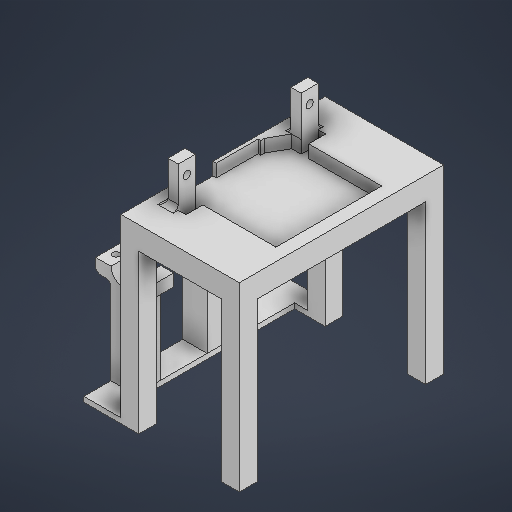
# Autodesk Inventor part: OMG_20kg_servo_side_profile(0.4mm)
Saved by Autodesk Inventor 2026.1 (Build 301233020, 233B)
## iProperties
Created: 2026-02-21
Part Number: OMG_20kg_servo_side_profile(0.4mm)
Material: Generic
Document SubType Name: Modeling
Designer: Lars
Density: 1 g/cm^3
Appearance: Default
Author: Lars
Autodesk Inventor part; units mm, degrees
ref_plane "YZ Plane" through (0, 0, 0) normal (1, 0, 0) x (0, 1, 0)
ref_plane "XZ Plane" through (0, 0, 0) normal (0, 1, 0) x (-1, 0, 0)
ref_plane "XY Plane" through (0, 0, 0) normal (0, 0, 1) x (1, 0, 0)
sketch "Sketch1" plane through (0, 0, 0) normal (0, 1, 0) x (-1, 0, 0)
  line L0 (0, 0) -> (28.63, 0)
  line L1 (28.63, 0) -> (28.63, -41.25) construction
  line L2 (28.63, -41.25) -> (0, -41.25)
  line L3 (0, -41.25) -> (0, 0)
  line L4 (28.63, 6.675) -> (31.43, 6.675)
  line L5 (31.43, 6.675) -> (31.43, 0)
  line L6 (31.43, -47.925) -> (28.63, -47.925)
  line L7 (28.63, -47.925) -> (28.63, -41.25)
  line L8 (31.43, -20.625) -> (28.63, -20.625) construction
  line L9 (38.98, 0) -> (31.43, 0)
  line L10 (31.43, 0) -> (31.43, -41.25) construction
  line L11 (31.43, -41.25) -> (35.18, -41.25)
  line L12 (38.98, -41.25) -> (38.98, -34.5) construction
  line L13 (31.43, -41.25) -> (35.18, -41.25) construction
  line L14 (38.98, 0) -> (38.98, -1) construction
  line L15 (38.98, -34.5) -> (35.18, -41.25)
  line L16 (38.98, -34.5) -> (38.98, -33)
  line L17 (35.18, -41.25) -> (38.98, -41.25) construction
  line L18 (38.98, 0) -> (38.98, -1) construction
  line L19 (38.98, -1) -> (39.98, -1)
  line L20 (39.98, -1) -> (39.98, -4)
  line L21 (39.98, -33) -> (38.98, -33)
  line L22 (38.98, -33) -> (38.98, -1) construction
  line L23 (38.98, -1) -> (38.98, -33) construction
  line L24 (38.98, -33) -> (38.98, -34.5) construction
  line L25 (38.98, -1) -> (38.98, 0)
  line L26 (38.98, -33) -> (38.98, -1) construction
  line L27 (31.43, 0) -> (31.43, -41.25) construction
  line L28 (31.43, -41.25) -> (31.43, -47.925)
  line L29 (28.63, -41.25) -> (28.63, 0) construction
  line L30 (28.63, 0) -> (28.63, 6.675)
  line L31 (28.63, 0) -> (31.43, 0) construction
  line L32 (31.43, -41.25) -> (28.63, -41.25) construction
  line L33 (39.98, -1) -> (39.98, -4) construction
  line L34 (39.98, -4) -> (41.28, -4)
  line L35 (41.28, -4) -> (41.28, -16.6)
  line L36 (41.28, -16.6) -> (39.98, -16.6)
  line L37 (39.98, -16.6) -> (39.98, -4) construction
  line L38 (39.98, -4) -> (39.98, -16.6) construction
  line L39 (39.98, -16.6) -> (39.98, -33)
  line L40 (41.38, -16.7) -> (41.38, -3.9)
  line L41 (41.38, -3.9) -> (40.08, -3.9)
  line L42 (40.08, -3.9) -> (40.08, -0.9)
  line L43 (40.08, -0.9) -> (39.08, -0.9)
  line L44 (39.08, -0.9) -> (39.08, 0.1)
  line L45 (39.08, 0.1) -> (31.53, 0.1)
  line L46 (31.53, 0.1) -> (31.53, 6.775)
  line L47 (31.53, 6.775) -> (28.53, 6.775)
  line L48 (28.53, 6.775) -> (28.53, 0.1)
  line L49 (28.53, 0.1) -> (-0.1, 0.1)
  line L50 (-0.1, 0.1) -> (-0.1, -41.35)
  line L51 (-0.1, -41.35) -> (28.53, -41.35)
  line L52 (28.53, -41.35) -> (28.53, -48.025)
  line L53 (28.53, -48.025) -> (31.53, -48.025)
  line L54 (31.53, -48.025) -> (31.53, -41.35)
  line L55 (31.53, -41.35) -> (35.2385, -41.35)
  line L56 (35.2385, -41.35) -> (39.08, -34.5262)
  line L57 (39.08, -34.5262) -> (39.08, -33.1)
  line L58 (39.08, -33.1) -> (40.08, -33.1)
  line L59 (40.08, -33.1) -> (40.08, -16.7)
  line L60 (40.08, -16.7) -> (41.38, -16.7)
  line L61 (0, -20.625) -> (39.98, -20.625) construction
  line L62 (44.99, 9.375) -> (-5.01, 9.375)
  line L63 (-5.01, 9.375) -> (-5.01, -50.625)
  line L64 (-5.01, -50.625) -> (44.99, -50.625)
  line L65 (44.99, -50.625) -> (44.99, 9.375)
  line L66 (19.99, 9.375) -> (19.99, -50.625) construction
  point P0 (30.03, 6.675)
  point P1 (19.99, -20.625)
  dimension "d0" = 28.63
  dimension "d1" = 41.25
  dimension "d2" = 2.8
  dimension "d3" = 54.6
  dimension "d4" = 7.55
  dimension "d5" = 41.25
  dimension "d6" = 3.75
  dimension "d7" = 34.5
  dimension "d8" = 1
  dimension "d9" = 32
  dimension "d10" = 1
  dimension "d11" = 6.675
  dimension "d12" = 3
  dimension "d13" = 1.3
  dimension "d14" = 12.6
  dimension "d15" = 0.1
  dimension "d16" = 50
  dimension "d17" = 60
  constraints: 134 end point, 35 parallel, 17 perpendicular, 8 midpoint, 7 horizontal, 5 vertical, 1 point on line, 20 other
  measures "d0" distance of L1.end L2.end
  measures "d1" distance of L0.end L1.end
  measures "d2" distance of L6.start L6.end
  measures "d3" distance of L4.end L6.start
  measures "d4" distance of L12.start L10.end
  measures "d5" distance of L12.start L9.start
  measures "d6" distance of L10.end L11.end
  measures "d7" distance of L9.start L12.end
  measures "d8" distance of L9.start L14.end
  measures "d9" distance of L19.end L21.start
  measures "d10" distance of L21.start L16.end
  measures "d11" distance from line of point (30.03, 6.675) L31
  measures "d12" distance of L19.end L20.end
  measures "d13" distance of L35.end L36.end
  measures "d14" distance of L34.end L35.end
  measures "d15" distance between parallel lines of L35 L40
  measures "d16" distance of L64.end L63.end
  measures "d17" distance of L63.end L62.end
extrude "Extrusion1" add sketch "Sketch1" along normal blind 5 contours L65 L64 L63 L62
sketch "Sketch3" plane through (5.01, 0, -50.625) normal (0, 0, -1) x (-1, 0, 0)
  line L0 (0, 5) -> (50, 5) projected
  line L1 (0, 0) -> (50, 0) projected
  line L2 (0, 5) -> (50, 5)
  line L3 (50, 5) -> (50, 0)
  line L4 (50, 0) -> (0, 0)
  line L5 (0, 0) -> (0, 5)
  point P0 (5.01, 0)
  constraints: 8 end point, 2 parallel, 1 horizontal, 1 perpendicular
sketch "Sketch4" plane through (-44.99, 0, 9.375) normal (0, 0, 1) x (1, 0, 0)
  line L0 (0, 0) -> (0, 5) projected
  line L1 (50, 0) -> (0, 0) projected
  line L2 (0, 5) -> (50, 5)
  line L3 (50, 5) -> (50, 0)
  line L4 (50, 0) -> (0, 0)
  line L5 (0, 0) -> (0, 5)
  point P0 (44.99, 0)
  constraints: 8 end point, 2 parallel, 1 horizontal, 1 perpendicular
extrude "Extrusion2" add sketch "Sketch4" along normal blind 10
extrude "Extrusion3" add sketch "Sketch3" along normal blind 10
sketch "Sketch5" plane through (0, 5, 0) normal (0, 1, 0) x (1, 0, 0)
  line L0 (-41.38, 3.9) -> (-41.38, 16.7) projected
  line L1 (-44.99, -19.375) -> (-44.99, 60.625) projected
  line L2 (-44.99, 16.7) -> (-44.99, -19.375)
  line L3 (-44.99, -19.375) -> (-41.38, -19.375)
  line L4 (-41.38, -19.375) -> (-41.38, 16.7)
  line L5 (-44.99, 60.625) -> (-41.38, 60.625)
  line L6 (-41.38, 60.625) -> (-41.38, 16.7)
  line L7 (-44.99, 16.7) -> (-44.99, 60.625)
  point P0 (0, 0)
  constraints: 12 end point, 2 parallel, 1 horizontal, 1 perpendicular
extrude "Extrusion4" cut sketch "Sketch5" against normal blind 10
sketch "Sketch6" plane through (0, 0, 0) normal (0, -1, 0) x (1, 0, 0)
  line L0 (5.01, -60.625) -> (5.01, 19.375) projected
  line L1 (5.01, 19.375) -> (-41.3631, 19.375)
  line L2 (-41.3631, 19.375) -> (-41.3631, -60.625)
  line L3 (-41.3631, -60.625) -> (5.01, -60.625)
  line L4 (5.01, -60.625) -> (5.01, 19.375)
  point P0 (0, 0)
  constraints: 8 end point, 2 parallel, 1 horizontal, 1 perpendicular
extrude "Extrusion5" add sketch "Sketch6" along normal blind 4
sketch "Sketch7" plane through (0, 5, 0) normal (0, 1, 0) x (1, 0, 0)
  line L0 (-31.53, -0.1) -> (-39.08, -0.1) projected
  line L1 (-31.53, -0.1) -> (-35.53, -0.1)
  line L2 (-35.53, -0.1) -> (-35.53, -6.775)
  line L3 (-35.53, -6.775) -> (-31.53, -6.775)
  line L4 (-31.53, -6.775) -> (-31.53, -0.1)
  line L5 (-31.53, 41.3538) -> (-35.53, 41.3538)
  line L6 (-35.53, 41.3538) -> (-35.53, 48.025)
  line L7 (-35.53, 48.025) -> (-31.53, 48.025)
  line L8 (-31.53, 48.025) -> (-31.53, 41.3538)
  point P0 (0, 0)
  dimension "d28" = 4
  dimension "d29" = 4
  constraints: 16 end point, 4 parallel, 2 horizontal, 2 perpendicular, 1 point on line
  measures "d28" distance of L3.end L2.end
  measures "d29" distance of L6.end L7.end
extrude "Extrusion6" add sketch "Sketch7" along normal blind 15.7
sketch "Sketch8" plane through (-35.53, 5, 0.1) normal (-1, 0, 0) x (0, 0, 1)
  line L0 (6.675, 15.7) -> (0, 15.7) projected
  line L1 (3.3375, 15.7) -> (3.3375, 10.325) construction
  line L2 (-41.4538, 15.7) -> (-48.125, 15.7) projected
  line L3 (-44.7894, 15.7) -> (-44.7894, 10.325) construction
  circle A0 centre (-44.7894, 10.325) radius 1.45
  circle A1 centre (3.3375, 10.325) radius 1.45
  point P0 (-0.1, -5)
  dimension "d32" = 5.375
  dimension "d33" = 5.375
  dimension "d34" = 2.9
  dimension "d35" = 2.9
  constraints: 4 end point, 2 centre point, 2 coincident, 2 midpoint, 2 vertical
  measures "d32" distance of L1.start L1.end
  measures "d33" distance of L3.start L3.end
  measures "d34" diameter of A0
  measures "d35" diameter of A1
extrude "Extrusion7" cut sketch "Sketch8" against normal through all
fillet "Fillet1" radius 2 4 edges at (-35.53, 5, -44.6894) (-35.53, 5, 3.4375) (-33.53, 5, 6.775) (-33.53, 5, -48.025)
sketch "Sketch9" plane through (0, -4, 0) normal (0, -1, 0) x (1, 0, 0)
  line L0 (-41.38, -60.625) -> (5.01, -60.625) projected
  line L1 (-41.38, -60.625) -> (-34.38, -60.625)
  line L2 (-34.38, -60.625) -> (-34.38, -53.625)
  line L3 (-34.38, -53.625) -> (-41.38, -53.625)
  line L4 (-41.38, -53.625) -> (-41.38, -60.625)
  line L5 (5.01, -60.625) -> (-1.99, -60.625)
  line L6 (-1.99, -60.625) -> (-1.99, -53.625)
  line L7 (-1.99, -53.625) -> (5.01, -53.625)
  line L8 (5.01, -53.625) -> (5.01, -60.625)
  line L9 (5.01, 19.375) -> (-41.38, 19.375) projected
  line L10 (5.01, 19.375) -> (-1.99, 19.375)
  line L11 (-1.99, 19.375) -> (-1.99, 12.375)
  line L12 (-1.99, 12.375) -> (5.01, 12.375)
  line L13 (5.01, 12.375) -> (5.01, 19.375)
  line L14 (-41.38, 19.375) -> (-34.38, 19.375)
  line L15 (-34.38, 19.375) -> (-34.38, 12.375)
  line L16 (-34.38, 12.375) -> (-41.38, 12.375)
  line L17 (-41.38, 12.375) -> (-41.38, 19.375)
  point P0 (0, 0)
  dimension "d39" = 7
  dimension "d40" = 7
  dimension "d41" = 7
  dimension "d42" = 7
  dimension "d43" = 7
  dimension "d44" = 7
  dimension "d45" = 7
  dimension "d46" = 7
  constraints: 32 end point, 8 parallel, 4 horizontal, 4 perpendicular
  measures "d39" distance of L3.end L2.end
  measures "d40" distance of L2.end L1.end
  measures "d41" distance of L6.end L7.end
  measures "d42" distance of L5.end L6.end
  measures "d43" distance of L12.end L11.end
  measures "d44" distance of L11.end L10.end
  measures "d45" distance of L15.end L16.end
  measures "d46" distance of L14.end L15.end
extrude "Extrusion8" add sketch "Sketch9" along normal blind 60
sketch "Sketch10" plane through (0, -64, 0) normal (0, -1, 0) x (1, 0, 0)
  line L0 (5.01, -60.625) -> (5.01, 19.375) projected
  line L1 (5.01, 19.375) -> (-54.99, 19.375)
  line L2 (-54.99, 19.375) -> (-54.99, -60.625)
  line L3 (-54.99, -60.625) -> (5.01, -60.625)
  line L4 (5.01, -60.625) -> (5.01, 19.375)
  point P0 (0, 0)
  dimension "d49" = 60
  constraints: 8 end point, 2 parallel, 1 horizontal, 1 perpendicular
  measures "d49" distance of L3.end L2.end
extrude "Extrusion9" add sketch "Sketch10" along normal blind 2
sketch "Sketch12" plane through (0, -64, 0) normal (0, 1, 0) x (1, 0, 0)
  line L0 (-41.3631, 3.9) -> (-41.3631, 16.7) projected
  line L1 (-41.3631, 10.3) -> (-46.3231, 10.3) construction
  line L2 (-46.3231, 10.3) -> (-46.3231, 1.25) construction
  line L3 (-46.3231, 10.3) -> (-46.3231, 19.35) construction
  line L4 (-46.3231, 1.25) -> (-55.9231, 1.25)
  line L5 (-55.9231, 1.25) -> (-55.9231, -8.75)
  line L6 (-55.9231, -8.75) -> (-46.3231, -8.75)
  line L7 (-46.3231, -8.75) -> (-46.3231, 1.25)
  line L8 (-46.3231, 19.35) -> (-55.9231, 19.35)
  line L9 (-55.9231, 19.35) -> (-55.9231, 29.35)
  line L10 (-55.9231, 29.35) -> (-46.3231, 29.35)
  line L11 (-46.3231, 29.35) -> (-46.3231, 19.35)
  point P0 (0, 0)
  dimension "d52" = 4.96
  dimension "d53" = 9.05
  dimension "d54" = 9.05
  dimension "d55" = 9.6
  dimension "d56" = 10
  dimension "d57" = 9.6
  dimension "d58" = 10
  constraints: 22 end point, 4 parallel, 3 horizontal, 2 perpendicular, 2 vertical, 1 midpoint
  measures "d52" distance of L1.start L1.end
  measures "d53" distance of L1.end L2.end
  measures "d54" distance of L1.end L3.end
  measures "d55" distance of L6.end L5.end
  measures "d56" distance of L5.end L4.end
  measures "d57" distance of L9.end L10.end
  measures "d58" distance of L8.end L9.end
extrude "Extrusion10" add sketch "Sketch12" along normal blind 38.85
sketch "Sketch14" plane through (-55.9231, -64, -29.35) normal (-1, 0, 0) x (0, 0, 1)
  line L0 (0, 0) -> (0, 38.85) projected
  line L1 (10, 0) -> (10, 38.85) projected
  line L2 (0, 38.85) -> (10, 38.85)
  line L3 (10, 38.85) -> (10, 33.85)
  line L4 (10, 33.85) -> (0, 33.85)
  line L5 (0, 33.85) -> (0, 38.85)
  line L6 (28.1, 0) -> (28.1, 38.85) projected
  line L7 (38.1, 0) -> (38.1, 38.85) projected
  line L8 (28.1, 38.85) -> (38.1, 38.85)
  line L9 (38.1, 38.85) -> (38.1, 33.85)
  line L10 (38.1, 33.85) -> (28.1, 33.85)
  line L11 (28.1, 33.85) -> (28.1, 38.85)
  point P0 (29.35, 64)
  dimension "d61" = 5
  dimension "d62" = 5
  constraints: 16 end point, 4 parallel, 2 horizontal, 2 perpendicular, 2 point on line
  measures "d61" distance of L2.end L3.end
  measures "d62" distance of L8.end L9.end
extrude "Extrusion11" add sketch "Sketch14" along normal blind 6
sketch "Sketch15" plane through (-46.3231, -64, 8.75) normal (1, 0, 0) x (0, 0, -1)
  line L0 (0, 38.85) -> (10, 38.85) projected
  line L1 (10, 0) -> (10, 38.85) projected
  line L2 (0, 38.85) -> (10, 38.85)
  line L3 (10, 38.85) -> (10, 33.85)
  line L4 (10, 33.85) -> (0, 33.85)
  line L5 (0, 33.85) -> (0, 38.85)
  line L6 (28.1, 0) -> (28.1, 38.85) projected
  line L7 (38.1, 0) -> (38.1, 38.85) projected
  line L8 (28.1, 38.85) -> (38.1, 38.85)
  line L9 (38.1, 38.85) -> (38.1, 33.85)
  line L10 (38.1, 33.85) -> (28.1, 33.85)
  line L11 (28.1, 33.85) -> (28.1, 38.85)
  point P0 (8.75, 64)
  dimension "d65" = 5
  dimension "d66" = 5
  constraints: 16 end point, 4 parallel, 2 horizontal, 2 perpendicular, 2 point on line
  measures "d65" distance of L2.end L3.end
  measures "d66" distance of L8.end L9.end
extrude "Extrusion12" add sketch "Sketch15" along normal blind 6
sketch "Sketch16" plane through (-46.3231, -64, -29.35) normal (0, 0, -1) x (-1, 0, 0)
  line L0 (-6, 38.85) -> (15.6, 38.85) projected
  circle A0 centre (4.8, 38.85) radius 4.75
  point P0 (-46.3231, 64)
  dimension "d69" = 9.5
  constraints: 1 centre point, 1 midpoint
  measures "d69" diameter of A0
extrude "Extrusion13" cut sketch "Sketch16" against normal through all
sketch "Sketch17" plane through (0, -25.15, 0) normal (0, 1, 0) x (1, 0, 0)
  circle A0 centre (-58.923, 24.35) radius 1.35
  circle A1 centre (-58.923, -3.75) radius 1.35
  point P0 (0, 0)
  dimension "d72" = 2.7
  dimension "d73" = 2.7
  constraints: 2 centre point
  measures "d72" diameter of A0
  measures "d73" diameter of A1
extrude "Extrusion14" cut sketch "Sketch17" against normal through all
fillet "Fillet2" radius 2 8 edges at (-55.9231, -30.15, 3.75) (-55.9231, -30.15, -24.35) (-46.3231, -30.15, 3.75) (-46.3231, -30.15, -24.35) (-61.9231, -30.15, -24.35) (-61.9231, -30.15, 3.75) (-40.3231, -30.15, -24.35) (-40.3231, -30.15, 3.75)
sketch "Sketch18" plane through (0, -66, 0) normal (0, -1, 0) x (1, 0, 0)
  line L0 (5.01, 19.375) -> (-54.99, 19.375) projected
  line L1 (-54.99, 19.375) -> (-55.923, 19.375)
  line L2 (-55.923, 19.375) -> (-55.923, -60.625)
  line L3 (-55.923, -60.625) -> (-54.99, -60.625)
  line L4 (-54.99, -60.625) -> (-54.99, 19.375)
  point P0 (0, 0)
  dimension "d77" = 0.933
  constraints: 8 end point, 2 parallel, 1 horizontal, 1 perpendicular
  measures "d77" distance of L3.end L2.end
extrude "Extrusion15" add sketch "Sketch18" against normal blind 2
sketch "Sketch19" plane through (0, -64, 0) normal (0, 1, 0) x (1, 0, 0)
  line L0 (5.01, 53.625) -> (-1.99, 53.625) projected
  line L1 (-46.323, 53.625) -> (-46.323, -12.375)
  line L2 (5.01, -12.375) -> (5.01, 53.625)
  line L3 (-1.99, -19.375) -> (-1.99, -12.375) projected
  line L4 (-1.99, -12.375) -> (-1.99, -19.375)
  line L5 (-1.99, -19.375) -> (-34.38, -19.375)
  line L6 (-34.38, -12.375) -> (-34.38, -19.375) projected
  line L7 (-34.38, -19.375) -> (-34.38, -12.375)
  line L8 (-46.323, -12.375) -> (-34.38, -12.375)
  line L9 (-1.99, -12.375) -> (5.01, -12.375)
  line L10 (-34.38, 60.625) -> (-34.38, 53.625) projected
  line L11 (-34.38, 53.625) -> (-34.38, 60.625)
  line L12 (-1.99, 53.625) -> (-1.99, 60.625) projected
  line L13 (-34.38, 60.625) -> (-1.99, 60.625)
  line L14 (-1.99, 60.625) -> (-1.99, 53.625)
  line L15 (5.01, 53.625) -> (-1.99, 53.625)
  line L16 (-34.38, 53.625) -> (-46.323, 53.625)
  point P0 (0, 0)
  dimension "d81" = 51.333
  constraints: 24 end point, 6 perpendicular, 5 parallel, 3 collinear, 2 horizontal
  measures "d81" distance of L2.start L1.end
extrude "Extrusion16" cut sketch "Sketch19" against normal through all
sketch "Sketch21" plane through (0, -25.15, 0) normal (0, 1, 0) x (1, 0, 0)
  line L0 (-40.3231, -8.75) -> (-46.3731, -8.75) projected
  line L1 (-42.3231, 29.35) -> (-40.3231, 29.35) projected
  line L2 (-41.3631, -8.75) -> (-40.3231, -8.75)
  line L3 (-40.3231, -8.75) -> (-40.3231, 29.35)
  line L4 (-40.3231, 29.35) -> (-41.3631, 29.35)
  line L5 (-41.3631, 29.35) -> (-41.3631, -8.75)
  point P0 (0, 0)
  constraints: 8 end point, 2 parallel, 1 horizontal, 1 perpendicular, 1 point on line
extrude "Extrusion17" cut sketch "Sketch21" against normal blind 6
equation "\"d5\" = d1"
body "Solid1"
